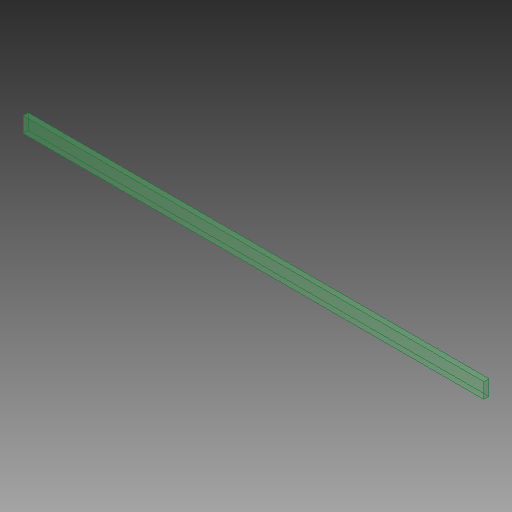
# Autodesk Inventor part: sb_support_side
Saved by Autodesk Inventor 2018.1 (Build 221171000, 171)
## iProperties
Created: 2017-08-17
Part Number: sb_support_side
Material: PVC-Piping
Document SubType Name: Modeling
Designer: Tom
Density: 1.4 g/cm^3
Appearance: Clear - Green 1
Author: Tom
Autodesk Inventor part; units mm, degrees
ref_plane "YZ Plane" through (0, 0, 0) normal (1, 0, 0) x (0, 1, 0)
ref_plane "XZ Plane" through (0, 0, 0) normal (0, 1, 0) x (-1, 0, 0)
ref_plane "XY Plane" through (0, 0, 0) normal (0, 0, 1) x (1, 0, 0)
sketch "Sketch2" plane through (0, 0, 0) normal (0, 0, 1) x (1, 0, 0)
  line L0 (-224.5, -7.5) -> (224.5, -7.5)
  line L1 (224.5, -7.5) -> (224.5, 7.5)
  line L2 (224.5, 7.5) -> (-224.5, 7.5)
  line L3 (-224.5, 7.5) -> (-224.5, -7.5)
  line L4 (-224.5, -7.5) -> (224.5, 7.5) construction
  line L5 (224.5, -7.5) -> (-224.5, 7.5) construction
  point P0 (0, 0)
  dimension "d4" = 449
  dimension "d5" = 15
  constraints: 12 end point, 2 midpoint, 2 parallel, 1 horizontal, 1 perpendicular
  measures "d4" distance of L2.end L1.end
  measures "d5" distance of L1.end L0.end
extrude "Extrusion2" add sketch "Sketch2" along normal mid plane 5
equation "\"d4\" = boxw - 2 * play"
equation "\"d5\" = supporth"
equation "\"d6\" = pvct"
equation "\"solhole\" = 3"
equation "\"solholespacing\" = 16"
equation "\"ssolw\" = 63"
equation "\"bsoll\" = 126"
equation "\"bsolw\" = 91"
equation "\"bsolh\" = 126"
equation "\"tapl\" = 31"
equation "\"tl\" = 32"
equation "\"eloboww\" = 25"
equation "\"pvct\" = 5"
equation "\"boxh\" = 258"
equation "\"supporth\" = 15"
equation "\"play\" = 0.5"
equation "\"pcbh\" = 46"
equation "\"pcbw\" = 76"
equation "\"arw\" = 54"
equation "\"arl\" = 102"
equation "\"pcbl\" = 86"
equation "\"psuh\" = 85"
equation "\"screenw\" = 197"
equation "\"screenl\" = 115"
equation "\"seph\" = 105"
equation "\"diapower\" = 16"
equation "\"distbubblewater\" = 82"
equation "\"distpumps\" = 75"
equation "\"pumpinner\" = 16"
equation "\"waterouter\" = 39"
equation "\"waterinner\" = 28"
equation "\"pumpouter\" = 25"
equation "\"airininner\" = 28"
equation "\"airoutinner\" = 28"
equation "\"airoutouter\" = 39"
equation "\"airinouter\" = 39"
equation "\"dialoadouter\" = 25"
equation "\"diaetapeouter\" = 36"
equation "\"diaetape\" = 25"
equation "\"diapowerouter\" = 25"
equation "\"diaphouter\" = 48"
equation "\"diaph\" = 32"
equation "\"diaload\" = 16"
equation "\"boxw\" = 450"
body "Solid2"
